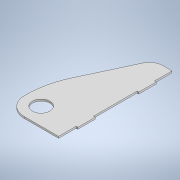
# Autodesk Inventor part: Beslag_stempel
Saved by Autodesk Inventor 2022 (Build 260153000, 153)
## iProperties
Created: 2022-04-09
Part Number: Beslag_stempel
Material: Generic
Document SubType Name: Sheet Metal
Designer: Patrick
Density: 1 g/cm^3
Sheet Metal Rule: Default_mm
Appearance: Default
Author: Patrick
Autodesk Inventor part; units mm, degrees
ref_plane "YZ Plane" through (0, 0, 0) normal (1, 0, 0) x (0, 1, 0)
ref_plane "XZ Plane" through (0, 0, 0) normal (0, 1, 0) x (-1, 0, 0)
ref_plane "XY Plane" through (0, 0, 0) normal (0, 0, 1) x (1, 0, 0)
sketch "Sketch1" plane through (0, 0, 0) normal (0, 1, 0) x (-1, 0, 0)
  line L0 (0, 0) -> (60, 0)
  line L1 (60, 0) -> (60, -45)
  line L2 (60, -45) -> (20.3638, -130)
  line L3 (20.3638, -130) -> (0, -130)
  line L4 (0, 0) -> (0, -130)
  circle A0 centre (40, -20) radius 10
  line L5 (0, -20) -> (-2, -20)
  line L6 (-2, -20) -> (-2, -40)
  line L7 (-2, -40) -> (0, -40)
  line L8 (0, -40) -> (0, -20)
  line L9 (0, -90) -> (-2, -90)
  line L10 (-2, -90) -> (-2, -110)
  line L11 (-2, -110) -> (0, -110)
  line L12 (0, -110) -> (0, -90)
  dimension "d0" = 45
  dimension "d1" = 40
  dimension "d2" = 20
  dimension "d3" = 20
  dimension "d4" = 130
  dimension "d5" = 20
  dimension "d10" = 25
  dimension "d11" = 2
  dimension "d12" = 2
  dimension "d13" = 20
  dimension "d14" = 20
  dimension "d15" = 20
  dimension "d16" = 20
  measures "d0" distance of L0.end L1.end
  measures "d1" distance from line of L4 A0.centre
  measures "d2" distance from line of A0.centre L0
  measures "d3" distance from line of L1 A0.centre
  measures "d4" distance of L0.start L3.end
  measures "d5" diameter of A0
  measures "d10" angle of L4 L2
  measures "d11" distance between parallel lines of L4 L6
  measures "d12" distance between parallel lines of L4 L10
  measures "d13" distance of L5.end L6.end
  measures "d14" distance of L9.end L10.end
  measures "d15" distance between parallel lines of L0 L5
  measures "d16" distance between parallel lines of L3 L11
extrude "Plate1" add sketch "Sketch1" along normal blind 2
fillet "Fillet1" radius 20.5 1 edges at (-60, 1, 0)
fillet "Fillet2" radius 103.25 1 edges at (-60, 1, -45)
fillet "Fillet3" radius 15.5 1 edges at (-20.3638, 1, -130)
equation "\"d6\" = Thickness"
equation "\"BendRadius\" = Thickness"
equation "\"BendReliefWidth\" = Thickness"
equation "\"BendReliefDepth\" = 0.5 * Thickness"
equation "\"CornerReliefSize\" = 4 * Thickness"
equation "\"MinimumRemnant\" = 2 * Thickness"
equation "\"TransitionRadius\" = BendRadius"
equation "\"JacobiRadiusSize\" = BendRadius"
equation "\"GapSize\" = Thickness"
equation "\"Thickness\" = 2"
body "Solid1"
